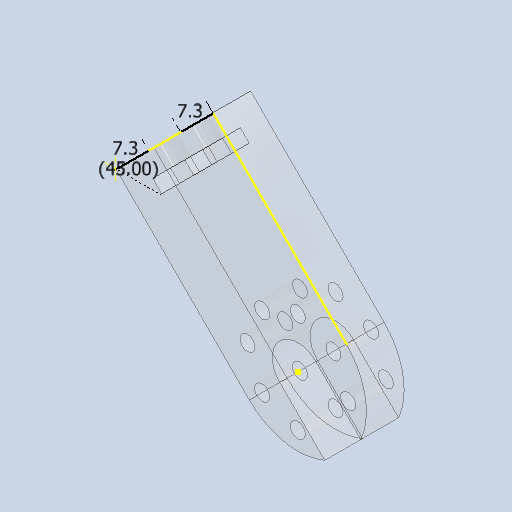
# Autodesk Inventor part: _armpit_adt_1
Saved by Autodesk Inventor 2024.3 (Build 283343000, 343)
## iProperties
Created: 2024-09-06
Part Number: _armpit_adt_1
Material: PMMA 플라스틱
Document SubType Name: Modeling
Designer: gretc
Density: 1.188 g/cm^3
Appearance: 폴리카보네이트 - 선명
Mass: 4.81321 g
Surface Area: 26.9487 cm^2
Volume: 4.05153 cm^3
Author: gretc
Autodesk Inventor part; units mm, degrees
ref_plane "YZ Plane" through (0, 0, 0) normal (1, 0, 0) x (0, 1, 0)
ref_plane "XZ Plane" through (0, 0, 0) normal (0, 1, 0) x (-1, 0, 0)
ref_plane "XY Plane" through (0, 0, 0) normal (0, 0, 1) x (1, 0, 0)
sketch "스케치1" plane through (0, 0, 0) normal (0, 0, 1) x (1, 0, 0)
  circle A0 centre (-5.6569, -5.6569) radius 1.2 projected
  circle A1 centre (5.6569, -5.6569) radius 1.2 projected
  circle A2 centre (5.6569, 5.6569) radius 1.2 projected
  circle A3 centre (-5.6569, 5.6569) radius 1.2 projected
  circle A4 centre (0, 0) radius 4 projected
  circle A5 centre (0, 0) radius 10.9 projected
  circle A6 centre (0, 8) radius 1.2 projected
  circle A7 centre (8, 0) radius 1.2 projected
  circle A8 centre (0, -8) radius 1.2 projected
  circle A9 centre (-8, 0) radius 1.2 projected
  circle A10 centre (0, 0) radius 4.05
  line L0 (-5.6569, -5.6569) -> (5.6569, 5.6569)
  line L1 (-2.8638, -2.8638) -> (2.8638, 2.8638)
  line L2 (2.8638, 2.8638) -> (13.4704, -7.7428)
  line L3 (13.4704, -7.7428) -> (7.7428, -13.4704)
  line L4 (7.7428, -13.4704) -> (-2.8638, -2.8638)
  line L5 (-5.6569, -5.6569) -> (-8.1671, -8.1671)
  line L6 (5.6569, 5.6569) -> (8.1671, 8.1671)
  line L7 (-7.7075, -7.7075) -> (7.7075, 7.7075)
  line L8 (7.7075, 7.7075) -> (-13.5057, 28.9207)
  line L9 (-13.5057, 28.9207) -> (-28.9207, 13.5057)
  line L10 (-28.9207, 13.5057) -> (-7.7075, -7.7075)
  point P0 (0, 0)
  point P1 (10.0195, -4.2919)
  point P2 (4.2919, -10.0195)
  dimension "d0" = 8.1
  dimension "d1" = 15
  dimension "d2" = 30
  constraints: 22 end point, 4 parallel, 4 point on circle, 4 point on line, 2 collinear, 2 perpendicular, 1 centre point, 1 coincident
  measures "d0" diameter of A10
  measures "d1" distance of L1.end L2.end
  measures "d2" distance of L8.end L7.end
extrude "돌출1" add sketch "스케치1" along normal blind 6 contours A0 L0 L4 A5 L5 | A0 L5 A5 L6 A2 L0 A10 | L10 L9 L8 A5 | L0 A2 L6 A5 L2
sketch "스케치3" plane through (0, 0, 6) normal (0, 0, 1) x (1, 0, 0)
  line L0 (-28.9207, 13.5057) -> (-23.7588, 18.6676)
  line L1 (-13.5057, 28.9207) -> (-28.9207, 13.5057) projected
  line L2 (-28.9207, 13.5057) -> (-21.6207, 13.5057) construction
  line L3 (7.7075, 7.7075) -> (-13.5057, 28.9207) projected
  line L4 (-13.5057, 28.9207) -> (-18.6676, 23.7588)
  point P0 (0, 0)
  dimension "d16" = 7.3
  dimension "d17" = 45
  dimension "d18" = 7.3
  constraints: 6 end point, 1 collinear, 1 equal length, 1 horizontal, 1 point on line
  measures "d16" distance of L0.start L0.end
  measures "d17" angle of L2 L0
  measures "d18" distance of L1.start L4.end
sketch "스케치4" plane through (-28.9207, 13.5057, 0) normal (-0.7071068, 0.7071068, 0) x (-0.7071068, -0.7071068, 0)
  line L0 (0, 6) -> (-7.3, 6) projected
  line L1 (-21.8, 6) -> (0, 6) projected
  line L2 (-21.8, 0) -> (0, 0) projected
  line L3 (0, 0) -> (0, 6) projected
  line L4 (-21.8, 6) -> (0, 6) projected
  line L5 (-21.8, 0) -> (-21.8, 6) projected
  line L6 (-21.8, 0) -> (-14.5, 0)
  line L7 (-14.5, 0) -> (-14.5, 6)
  line L8 (-14.5, 0) -> (-14.5, 6)
  line L9 (-14.5, 6) -> (-7.3, 6)
  line L10 (-7.3, 6) -> (-7.3, 0)
  line L11 (-7.3, 0) -> (-14.5, 0)
  line L12 (-14.5, 6) -> (-14.5, 3)
  line L13 (-7.3, 3) -> (-14.5, 3)
  circle A0 centre (-7.3, 3) radius 1.35
  circle A1 centre (-14.5, 3) radius 1.35
  point P0 (-10.9, 0)
  dimension "d19" = 7.3
  dimension "d20" = 2.7
  dimension "d21" = 2.7
  constraints: 16 end point, 4 perpendicular, 2 centre point, 2 coincident, 2 midpoint, 2 parallel, 2 point on line
  measures "d19" distance of L2.start L6.end
  measures "d20" diameter of A0
  measures "d21" diameter of A1
extrude "돌출3" cut sketch "스케치4" against normal blind 4 contours A0 L10 | L10 L13 A0 | A1 L13 L7 | L7 A1 | L10 A0 L13 | L13 A1 L7
sketch "스케치5" plane through (0, 0, 6) normal (0, 0, 1) x (1, 0, 0)
  line L0 (-21.885, 14.8846) -> (-19.9758, 16.7938) projected
  line L1 (-16.7938, 19.9758) -> (-14.8846, 21.885) projected
  line L2 (-18.809, 16.5463) -> (-20.2233, 17.9605)
  line L3 (-20.2233, 17.9605) -> (-23.0517, 15.1321)
  line L4 (-23.0517, 15.1321) -> (-21.6375, 13.7179)
  line L5 (-21.6375, 13.7179) -> (-18.809, 16.5463)
  line L6 (-18.809, 16.5463) -> (-23.0517, 15.1321) construction
  line L7 (-20.2233, 17.9605) -> (-21.6375, 13.7179) construction
  line L8 (-13.7179, 21.6375) -> (-15.1321, 23.0517)
  line L9 (-15.1321, 23.0517) -> (-17.9605, 20.2233)
  line L10 (-17.9605, 20.2233) -> (-16.5463, 18.809)
  line L11 (-16.5463, 18.809) -> (-13.7179, 21.6375)
  line L12 (-13.7179, 21.6375) -> (-17.9605, 20.2233) construction
  line L13 (-15.1321, 23.0517) -> (-16.5463, 18.809) construction
  point P0 (0, 0)
  point P1 (-20.9304, 15.8392)
  point P2 (-15.8392, 20.9304)
  dimension "d24" = 2
  dimension "d25" = 4
  dimension "d26" = 2
  dimension "d27" = 4
  constraints: 24 end point, 6 midpoint, 4 parallel, 3 perpendicular
  measures "d24" distance of L2.start L2.end
  measures "d25" distance of L3.end L2.end
  measures "d26" distance of L8.start L8.end
  measures "d27" distance of L9.end L8.end
extrude "돌출4" cut sketch "스케치5" against normal blind 6
